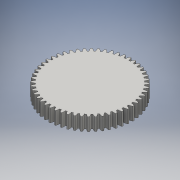
# Autodesk Inventor part: SUPERGEAR2
Saved by Autodesk Inventor 2016 (Build 200138000, 138)
## iProperties
Created: 2018-03-03
Part Number: SUPERGEAR2
Material: Generic
Document SubType Name: Modeling
Designer: Simon
Density: 1 g/cm^3
Appearance: Default
Author: Simon
Autodesk Inventor part; units mm, degrees
ref_plane "YZ Plane" through (0, 0, 0) normal (1, 0, 0) x (0, 1, 0)
ref_plane "XZ Plane" through (0, 0, 0) normal (0, 1, 0) x (-1, 0, 0)
ref_plane "XY Plane" through (0, 0, 0) normal (0, 0, 1) x (1, 0, 0)
sketch "Sketch1" plane through (0, 0, 0) normal (0, 0, 1) x (1, 0, 0)
  circle A0 centre (181.9844, -264.0466) radius 21.001
  arc A1 (180.8662, -241.2468) -> (180.3319, -243.1107) centre (187.0577, -244.0302) ccw
  arc A2 (182.1383, -243.0461) -> (181.4724, -241.2252) centre (175.4953, -244.4433) ccw
  line L0 (180.8662, -241.2468) -> (181.4724, -241.2252)
  arc A3 (182.1383, -243.0461) -> (180.3319, -243.1107) centre (181.9844, -264.0466) ccw
  line L1 (178.1262, -241.5478) -> (178.7253, -241.4533)
  arc A4 (178.1262, -241.5478) -> (177.8204, -243.4625) centre (184.608, -243.5646) ccw
  arc A5 (179.6059, -243.1807) -> (178.7253, -241.4533) centre (173.1797, -245.3684) ccw
  arc A6 (179.6059, -243.1807) -> (177.8204, -243.4625) centre (181.9844, -264.0466) ccw
  line L2 (175.4424, -242.1769) -> (176.0257, -242.0108)
  arc A7 (175.4424, -242.1769) -> (175.3697, -244.1145) centre (182.1201, -243.3977) ccw
  arc A8 (177.1081, -243.6195) -> (176.0257, -242.0108) centre (170.9925, -246.5659) ccw
  arc A9 (177.1081, -243.6195) -> (175.3697, -244.1145) centre (181.9844, -264.0466) ccw
  line L3 (172.854, -243.1249) -> (173.4131, -242.8897)
  arc A10 (172.854, -243.1249) -> (173.0153, -245.0571) centre (179.6301, -243.5319) ccw
  arc A11 (174.6815, -244.3562) -> (173.4131, -242.8897) centre (168.9656, -248.0183) ccw
  arc A12 (174.6815, -244.3562) -> (173.0153, -245.0571) centre (181.9844, -264.0466) ccw
  line L4 (170.3987, -244.378) -> (170.9254, -244.0771)
  arc A13 (170.3987, -244.378) -> (170.7918, -246.2767) centre (177.1745, -243.9652) ccw
  arc A14 (172.3613, -245.38) -> (170.9254, -244.0771) centre (167.1285, -249.7044) ccw
  arc A15 (172.3613, -245.38) -> (170.7918, -246.2767) centre (181.9844, -264.0466) ccw
  line L5 (168.1124, -245.9179) -> (168.599, -245.5558)
  arc A16 (168.1124, -245.9179) -> (168.7315, -247.7554) centre (174.7891, -244.6914) ccw
  arc A17 (170.1815, -246.6761) -> (168.599, -245.5558) centre (165.5081, -251.5996) ccw
  arc A18 (170.1815, -246.6761) -> (168.7315, -247.7554) centre (181.9844, -264.0466) ccw
  line L6 (166.0284, -247.7222) -> (166.4678, -247.304)
  arc A19 (166.0284, -247.7222) -> (166.8644, -249.4716) centre (172.5085, -245.6998) ccw
  arc A20 (168.1738, -248.2254) -> (166.4678, -247.304) centre (164.1279, -253.6764) ccw
  arc A21 (168.1738, -248.2254) -> (166.8644, -249.4716) centre (181.9844, -264.0466) ccw
  line L7 (164.177, -249.7645) -> (164.5628, -249.2964)
  arc A22 (164.177, -249.7645) -> (165.2179, -251.4004) centre (170.3662, -246.9758) ccw
  arc A23 (166.3674, -250.0054) -> (164.5628, -249.2964) centre (163.0081, -255.9043) ccw
  arc A24 (166.3674, -250.0054) -> (165.2179, -251.4004) centre (181.9844, -264.0466) ccw
  line L8 (162.5854, -252.015) -> (162.9119, -251.5039)
  arc A25 (162.5854, -252.015) -> (163.8158, -253.5135) centre (168.3932, -248.5007) ccw
  arc A26 (164.7888, -251.9902) -> (162.9119, -251.5039) centre (162.165, -258.251) ccw
  arc A27 (164.7888, -251.9902) -> (163.8158, -253.5135) centre (181.9844, -264.0466) ccw
  line L9 (161.2766, -254.4411) -> (161.5391, -253.8943)
  arc A28 (161.2766, -254.4411) -> (162.6786, -255.7803) centre (166.6185, -250.2522) ccw
  arc A29 (163.461, -254.1508) -> (161.5391, -253.8943) centre (161.611, -260.6823) ccw
  arc A30 (163.461, -254.1508) -> (162.6786, -255.7803) centre (181.9844, -264.0466) ccw
  line L10 (160.2697, -257.0071) -> (160.4644, -256.4327)
  arc A31 (160.2697, -257.0071) -> (161.823, -258.1676) centre (165.0678, -252.205) ccw
  arc A32 (162.4032, -256.4557) -> (160.4644, -256.4327) centre (161.354, -263.1625) ccw
  arc A33 (162.4032, -256.4557) -> (161.823, -258.1676) centre (181.9844, -264.0466) ccw
  line L11 (159.5796, -259.6759) -> (159.7036, -259.0821)
  arc A34 (159.5796, -259.6759) -> (161.2614, -260.6407) centre (163.7638, -254.3304) ccw
  arc A35 (161.631, -258.8713) -> (159.7036, -259.0821) centre (161.3978, -265.6557) ccw
  arc A36 (161.631, -258.8713) -> (161.2614, -260.6407) centre (181.9844, -264.0466) ccw
  line L12 (159.2161, -262.4083) -> (159.2676, -261.804)
  arc A37 (159.2161, -262.4083) -> (161.0019, -263.1634) centre (162.7255, -256.5975) ccw
  arc A38 (161.1556, -261.3624) -> (159.2676, -261.804) centre (161.7419, -268.1254) ccw
  arc A39 (161.1556, -261.3624) -> (161.0019, -263.1634) centre (181.9844, -264.0466) ccw
  line L13 (159.1846, -265.1647) -> (159.163, -264.5585)
  arc A40 (159.1846, -265.1647) -> (161.0485, -265.699) centre (161.968, -258.9732) ccw
  arc A41 (160.9839, -263.8926) -> (159.163, -264.5585) centre (162.3811, -270.5356) ccw
  arc A42 (160.9839, -263.8926) -> (161.0485, -265.699) centre (181.9844, -264.0466) ccw
  line L14 (159.4856, -267.9048) -> (159.3911, -267.3056)
  arc A43 (159.4856, -267.9048) -> (161.4003, -268.2105) centre (161.5024, -261.4229) ccw
  arc A44 (161.1185, -266.425) -> (159.3911, -267.3056) centre (163.3062, -272.8512) ccw
  arc A45 (161.1185, -266.425) -> (161.4003, -268.2105) centre (181.9844, -264.0466) ccw
  line L15 (160.1147, -270.5885) -> (159.9486, -270.0052)
  arc A46 (160.1147, -270.5885) -> (162.0523, -270.6613) centre (161.3355, -263.9108) ccw
  arc A47 (161.5573, -268.9228) -> (159.9486, -270.0052) centre (164.5037, -275.0384) ccw
  arc A48 (161.5573, -268.9228) -> (162.0523, -270.6613) centre (181.9844, -264.0466) ccw
  line L16 (161.0627, -273.1769) -> (160.8275, -272.6179)
  arc A49 (161.0627, -273.1769) -> (162.9949, -273.0156) centre (161.4697, -266.4008) ccw
  arc A50 (162.294, -271.3494) -> (160.8275, -272.6179) centre (165.9561, -277.0653) ccw
  arc A51 (162.294, -271.3494) -> (162.9949, -273.0156) centre (181.9844, -264.0466) ccw
  line L17 (162.3158, -275.6322) -> (162.015, -275.1055)
  arc A52 (162.3158, -275.6322) -> (164.2145, -275.2391) centre (161.903, -268.8564) ccw
  arc A53 (163.3178, -273.6696) -> (162.015, -275.1055) centre (167.6422, -278.9024) ccw
  arc A54 (163.3178, -273.6696) -> (164.2145, -275.2391) centre (181.9844, -264.0466) ccw
  line L18 (163.8557, -277.9185) -> (163.4936, -277.4319)
  arc A55 (163.8557, -277.9185) -> (165.6932, -277.2994) centre (162.6292, -271.2419) ccw
  arc A56 (164.6139, -275.8494) -> (163.4936, -277.4319) centre (169.5374, -280.5228) ccw
  arc A57 (164.6139, -275.8494) -> (165.6932, -277.2994) centre (181.9844, -264.0466) ccw
  line L19 (165.66, -280.0025) -> (165.2418, -279.5632)
  arc A58 (165.66, -280.0025) -> (167.4094, -279.1665) centre (163.6376, -273.5224) ccw
  arc A59 (166.1632, -277.8572) -> (165.2418, -279.5632) centre (171.6142, -281.903) ccw
  arc A60 (166.1632, -277.8572) -> (167.4094, -279.1665) centre (181.9844, -264.0466) ccw
  line L20 (167.7023, -281.8539) -> (167.2342, -281.4681)
  arc A61 (167.7023, -281.8539) -> (169.3382, -280.8131) centre (164.9136, -275.6648) ccw
  arc A62 (167.9432, -279.6635) -> (167.2342, -281.4681) centre (173.8421, -283.0228) ccw
  arc A63 (167.9432, -279.6635) -> (169.3382, -280.8131) centre (181.9844, -264.0466) ccw
  line L21 (169.9529, -283.4456) -> (169.4417, -283.119)
  arc A64 (169.9529, -283.4456) -> (171.4514, -282.2152) centre (166.4385, -277.6377) ccw
  arc A65 (169.928, -281.2421) -> (169.4417, -283.119) centre (176.1888, -283.8659) ccw
  arc A66 (169.928, -281.2421) -> (171.4514, -282.2152) centre (181.9844, -264.0466) ccw
  line L22 (172.3789, -284.7544) -> (171.8321, -284.4918)
  arc A67 (172.3789, -284.7544) -> (173.7181, -283.3523) centre (168.1901, -279.4125) ccw
  arc A68 (172.0886, -282.57) -> (171.8321, -284.4918) centre (178.6201, -284.42) ccw
  arc A69 (172.0886, -282.57) -> (173.7181, -283.3523) centre (181.9844, -264.0466) ccw
  line L23 (174.945, -285.7612) -> (174.3705, -285.5665)
  arc A70 (174.945, -285.7612) -> (176.1055, -284.2079) centre (170.1428, -280.9632) ccw
  arc A71 (174.3935, -283.6277) -> (174.3705, -285.5665) centre (181.1003, -284.6769) ccw
  arc A72 (174.3935, -283.6277) -> (176.1055, -284.2079) centre (181.9844, -264.0466) ccw
  line L24 (177.6137, -286.4514) -> (177.02, -286.3273)
  arc A73 (177.6137, -286.4514) -> (178.5785, -284.7695) centre (172.2682, -282.2672) ccw
  arc A74 (176.8091, -284.3999) -> (177.02, -286.3273) centre (183.5935, -284.6331) ccw
  arc A75 (176.8091, -284.3999) -> (178.5785, -284.7695) centre (181.9844, -264.0466) ccw
  line L25 (180.3462, -286.8148) -> (179.7418, -286.7633)
  arc A76 (180.3462, -286.8148) -> (181.1012, -285.029) centre (174.5353, -283.3055) ccw
  arc A77 (179.3002, -284.8753) -> (179.7418, -286.7633) centre (186.0632, -284.289) ccw
  arc A78 (179.3002, -284.8753) -> (181.1012, -285.029) centre (181.9844, -264.0466) ccw
  line L26 (183.1025, -286.8463) -> (182.4963, -286.868)
  arc A79 (183.1025, -286.8463) -> (183.6368, -284.9824) centre (176.911, -284.0629) ccw
  arc A80 (181.8304, -285.047) -> (182.4963, -286.868) centre (188.4734, -283.6498) ccw
  arc A81 (181.8304, -285.047) -> (183.6368, -284.9824) centre (181.9844, -264.0466) ccw
  line L27 (185.8426, -286.5453) -> (185.2434, -286.6399)
  arc A82 (185.8426, -286.5453) -> (186.1483, -284.6306) centre (179.3607, -284.5285) ccw
  arc A83 (184.3628, -284.9124) -> (185.2434, -286.6399) centre (190.789, -282.7247) ccw
  arc A84 (184.3628, -284.9124) -> (186.1483, -284.6306) centre (181.9844, -264.0466) ccw
  line L28 (188.5264, -285.9162) -> (187.943, -286.0823)
  arc A85 (188.5264, -285.9162) -> (188.5991, -283.9786) centre (181.8487, -284.6954) ccw
  arc A86 (186.8606, -284.4736) -> (187.943, -286.0823) centre (192.9762, -281.5272) ccw
  arc A87 (186.8606, -284.4736) -> (188.5991, -283.9786) centre (181.9844, -264.0466) ccw
  line L29 (191.1147, -284.9682) -> (190.5557, -285.2034)
  arc A88 (191.1147, -284.9682) -> (190.9534, -283.036) centre (184.3386, -284.5612) ccw
  arc A89 (189.2873, -283.7369) -> (190.5557, -285.2034) centre (195.0031, -280.0748) ccw
  arc A90 (189.2873, -283.7369) -> (190.9534, -283.036) centre (181.9844, -264.0466) ccw
  line L30 (193.57, -283.7151) -> (193.0433, -284.016)
  arc A91 (193.57, -283.7151) -> (193.1769, -281.8164) centre (186.7942, -284.1279) ccw
  arc A92 (191.6074, -282.7131) -> (193.0433, -284.016) centre (196.8402, -278.3887) ccw
  arc A93 (191.6074, -282.7131) -> (193.1769, -281.8164) centre (181.9844, -264.0466) ccw
  line L31 (195.8563, -282.1752) -> (195.3698, -282.5374)
  arc A94 (195.8563, -282.1752) -> (195.2372, -280.3378) centre (189.1797, -283.4017) ccw
  arc A95 (193.7873, -281.417) -> (195.3698, -282.5374) centre (198.4606, -276.4935) ccw
  arc A96 (193.7873, -281.417) -> (195.2372, -280.3378) centre (181.9844, -264.0466) ccw
  line L32 (197.9403, -280.3709) -> (197.501, -280.7891)
  arc A97 (197.9403, -280.3709) -> (197.1043, -278.6215) centre (191.4602, -282.3933) ccw
  arc A98 (195.795, -279.8677) -> (197.501, -280.7891) centre (199.8408, -274.4168) ccw
  arc A99 (195.795, -279.8677) -> (197.1043, -278.6215) centre (181.9844, -264.0466) ccw
  line L33 (199.7917, -278.3286) -> (199.4059, -278.7967)
  arc A100 (199.7917, -278.3286) -> (198.7509, -276.6928) centre (193.6026, -281.1173) ccw
  arc A101 (197.6013, -278.0877) -> (199.4059, -278.7967) centre (200.9606, -272.1888) ccw
  arc A102 (197.6013, -278.0877) -> (198.7509, -276.6928) centre (181.9844, -264.0466) ccw
  line L34 (201.3834, -276.0781) -> (201.0568, -276.5892)
  arc A103 (201.3834, -276.0781) -> (200.153, -274.5796) centre (195.5755, -279.5925) ccw
  arc A104 (199.1799, -276.1029) -> (201.0568, -276.5892) centre (201.8037, -269.8421) ccw
  arc A105 (199.1799, -276.1029) -> (200.153, -274.5796) centre (181.9844, -264.0466) ccw
  line L35 (202.6922, -273.6521) -> (202.4296, -274.1989)
  arc A106 (202.6922, -273.6521) -> (201.2901, -272.3128) centre (197.3503, -277.8409) ccw
  arc A107 (200.5078, -273.9423) -> (202.4296, -274.1989) centre (202.3578, -267.4109) ccw
  arc A108 (200.5078, -273.9423) -> (201.2901, -272.3128) centre (181.9844, -264.0466) ccw
  line L36 (203.699, -271.086) -> (203.5043, -271.6604)
  arc A109 (203.699, -271.086) -> (202.1457, -269.9255) centre (198.901, -275.8881) ccw
  arc A110 (201.5655, -271.6374) -> (203.5043, -271.6604) centre (202.6147, -264.9306) ccw
  arc A111 (201.5655, -271.6374) -> (202.1457, -269.9255) centre (181.9844, -264.0466) ccw
  line L37 (204.3892, -268.4172) -> (204.2651, -269.011)
  arc A112 (204.3892, -268.4172) -> (202.7074, -267.4524) centre (200.205, -273.7627) ccw
  arc A113 (202.3377, -269.2218) -> (204.2651, -269.011) centre (202.5709, -262.4374) ccw
  arc A114 (202.3377, -269.2218) -> (202.7074, -267.4524) centre (181.9844, -264.0466) ccw
  line L38 (204.7526, -265.6848) -> (204.7011, -266.2891)
  arc A115 (204.7526, -265.6848) -> (202.9668, -264.9297) centre (201.2433, -271.4956) ccw
  arc A116 (202.8131, -266.7307) -> (204.7011, -266.2891) centre (202.2268, -259.9677) ccw
  arc A117 (202.8131, -266.7307) -> (202.9668, -264.9297) centre (181.9844, -264.0466) ccw
  line L39 (204.7841, -262.9284) -> (204.8058, -263.5346)
  arc A118 (204.7841, -262.9284) -> (202.9203, -262.3941) centre (202.0007, -269.1199) ccw
  arc A119 (202.9848, -264.2005) -> (204.8058, -263.5346) centre (201.5876, -257.5575) ccw
  arc A120 (202.9848, -264.2005) -> (202.9203, -262.3941) centre (181.9844, -264.0466) ccw
  line L40 (204.4831, -260.1884) -> (204.5777, -260.7875)
  arc A121 (204.4831, -260.1884) -> (202.5684, -259.8826) centre (202.4663, -266.6702) ccw
  arc A122 (202.8502, -261.6681) -> (204.5777, -260.7875) centre (200.6625, -255.2419) ccw
  arc A123 (202.8502, -261.6681) -> (202.5684, -259.8826) centre (181.9844, -264.0466) ccw
  line L41 (203.854, -257.5046) -> (204.0201, -258.0879)
  arc A124 (203.854, -257.5046) -> (201.9164, -257.4319) centre (202.6332, -264.1823) ccw
  arc A125 (202.4114, -259.1703) -> (204.0201, -258.0879) centre (199.465, -253.0547) ccw
  arc A126 (202.4114, -259.1703) -> (201.9164, -257.4319) centre (181.9844, -264.0466) ccw
  line L42 (202.906, -254.9162) -> (203.1412, -255.4753)
  arc A127 (202.906, -254.9162) -> (200.9738, -255.0775) centre (202.499, -261.6923) ccw
  arc A128 (201.6747, -256.7437) -> (203.1412, -255.4753) centre (198.0127, -251.0278) ccw
  arc A129 (201.6747, -256.7437) -> (200.9738, -255.0775) centre (181.9844, -264.0466) ccw
  line L43 (201.6529, -252.4609) -> (201.9538, -252.9876)
  arc A130 (201.6529, -252.4609) -> (199.7542, -252.854) centre (202.0657, -259.2367) ccw
  arc A131 (200.6509, -254.4235) -> (201.9538, -252.9876) centre (196.3265, -249.1907) ccw
  arc A132 (200.6509, -254.4235) -> (199.7542, -252.854) centre (181.9844, -264.0466) ccw
  line L44 (200.113, -250.1746) -> (200.4752, -250.6612)
  arc A133 (200.113, -250.1746) -> (198.2756, -250.7937) centre (201.3395, -256.8513) ccw
  arc A134 (199.3549, -252.2437) -> (200.4752, -250.6612) centre (194.4313, -247.5703) ccw
  arc A135 (199.3549, -252.2437) -> (198.2756, -250.7937) centre (181.9844, -264.0466) ccw
  line L45 (198.3087, -248.0906) -> (198.7269, -248.5299)
  arc A136 (198.3087, -248.0906) -> (196.5593, -248.9266) centre (200.3311, -254.5707) ccw
  arc A137 (197.8055, -250.2359) -> (198.7269, -248.5299) centre (192.3546, -246.1901) ccw
  arc A138 (197.8055, -250.2359) -> (196.5593, -248.9266) centre (181.9844, -264.0466) ccw
  line L46 (196.2664, -246.2392) -> (196.7345, -246.625)
  arc A139 (196.2664, -246.2392) -> (194.6306, -247.2801) centre (199.0551, -252.4284) ccw
  arc A140 (196.0255, -248.4296) -> (196.7345, -246.625) centre (190.1266, -245.0703) ccw
  arc A141 (196.0255, -248.4296) -> (194.6306, -247.2801) centre (181.9844, -264.0466) ccw
  line L47 (194.0159, -244.6476) -> (194.527, -244.9741)
  arc A142 (194.0159, -244.6476) -> (192.5174, -245.878) centre (197.5303, -250.4554) ccw
  arc A143 (194.0407, -246.851) -> (194.527, -244.9741) centre (187.7799, -244.2272) ccw
  arc A144 (194.0407, -246.851) -> (192.5174, -245.878) centre (181.9844, -264.0466) ccw
  line L48 (191.5899, -243.3388) -> (192.1367, -243.6013)
  arc A145 (191.5899, -243.3388) -> (190.2506, -244.7408) centre (195.7787, -248.6807) ccw
  arc A146 (191.8801, -245.5232) -> (192.1367, -243.6013) centre (185.3487, -243.6732) ccw
  arc A147 (191.8801, -245.5232) -> (190.2506, -244.7408) centre (181.9844, -264.0466) ccw
  line L49 (189.0238, -242.3319) -> (189.5982, -242.5266)
  arc A148 (189.0238, -242.3319) -> (187.8633, -243.8852) centre (193.8259, -247.13) ccw
  arc A149 (189.5752, -244.4654) -> (189.5982, -242.5266) centre (182.8684, -243.4162) ccw
  arc A150 (189.5752, -244.4654) -> (187.8633, -243.8852) centre (181.9844, -264.0466) ccw
  line L50 (186.355, -241.6418) -> (186.9488, -241.7658)
  arc A151 (186.355, -241.6418) -> (185.3902, -243.3236) centre (191.7005, -245.826) ccw
  arc A152 (187.1596, -243.6932) -> (186.9488, -241.7658) centre (180.3752, -243.46) ccw
  arc A153 (187.1596, -243.6932) -> (185.3902, -243.3236) centre (181.9844, -264.0466) ccw
  line L51 (183.6226, -241.2783) -> (184.2269, -241.3298)
  arc A154 (183.6226, -241.2783) -> (182.8675, -243.0641) centre (189.4334, -244.7877) ccw
  arc A155 (184.6685, -243.2178) -> (184.2269, -241.3298) centre (177.9055, -243.8041) ccw
  arc A156 (184.6685, -243.2178) -> (182.8675, -243.0641) centre (181.9844, -264.0466) ccw
  point P0 (0, 0)
  dimension "d6" = 42.002
  dimension "d4" = 360
  constraints: 416 point on circle, 156 centre point, 104 end point, 681 other
extrude "Extrusion1" add sketch "Sketch1" along normal blind 7
body "Solid1"
